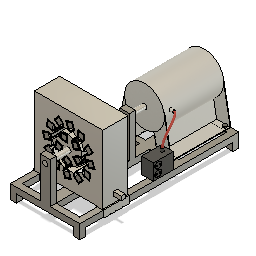
bannon_maher_magnetic_repulsion_motor_and_generator (Autodesk Fusion 360 design; units mm, degrees)
Autodesk Fusion 360 part; units mm, degrees
note: some values were not read from the file. Chosen so that the rebuilt part matches the saved one: which bodies a step acts on; which face or edge a step refers to. Set by a fixed rule: which sketch regions a step uses.
(part 1 of 2)
sketch "Sketch1" plane through (0, 0, 0) normal (0, 1, 0) x (1, 0, 0)
  line L0 (175, -400) -> (-175, -400)
  line L1 (-175, -400) -> (-175, 400)
  line L2 (-175, 400) -> (175, 400)
  line L3 (175, 400) -> (175, -400)
  line L4 (175, -400) -> (-175, 400) construction
  line L5 (-175, -400) -> (175, 400) construction
  line L6 (-145, -370) -> (-145, 370)
  line L7 (-145, 370) -> (145, 370)
  line L8 (145, 370) -> (145, -370)
  line L9 (145, -370) -> (-145, -370)
  dimension "d1" = 350
  dimension "d2" = 800
  dimension "d3" = 30
  measures "d1" distance of L1.end L2.end
  measures "d2" distance of L0.start L2.end
extrude "Extrude1" add sketch "Sketch1" along normal blind 30 makes body 1
sketch "Sketch2" plane through (0, 0, 0) normal (0, 1, 0) x (1, 0, 0)
  line L0 (-25, 370) -> (25, 370)
  line L1 (25, 370) -> (25, -370)
  line L2 (25, -370) -> (-25, -370)
  line L3 (-25, -370) -> (-25, 370)
  line L4 (-145, 370) -> (145, 370)
  line L5 (145, -370) -> (-145, -370)
  line L6 (0, 0) -> (0, 92.5114)
  dimension "d6" = 50
  measures "d6" distance of L1 L3
extrude "Extrude2" add sketch "Sketch2" along normal up to surface (30 mm away) bodies 1
ref_plane "WorkPlane1" through (0, 15, 400) normal (0, 0, -1) x (-1, 0, 0)
sketch "Sketch16" plane through (0, 0, 0) normal (0, -1, 0) x (1, 0, 0)
  line L0 (-25, -370) -> (-145, -370)
  line L1 (-145, -370) -> (-145, 370)
  line L2 (-145, 370) -> (-25, 370)
  line L3 (-25, 370) -> (-25, -370)
  line L4 (25, -370) -> (25, 370)
  line L5 (25, 370) -> (145, 370)
  line L6 (145, 370) -> (145, -370)
  line L7 (145, -370) -> (25, -370)
  line L8 (-175, -400) -> (175, -400)
  line L9 (175, -400) -> (175, 400)
  line L10 (175, 400) -> (-175, 400)
  line L11 (-175, 400) -> (-175, -400)
  line L12 (-175, 400) -> (-145, 400)
  line L13 (-145, 400) -> (-145, 370)
  line L14 (-145, 370) -> (-175, 370)
  line L15 (-175, 370) -> (-175, 400)
  line L16 (145, 370) -> (175, 370)
  line L17 (175, 370) -> (175, 400)
  line L18 (175, 400) -> (145, 400)
  line L19 (145, 400) -> (145, 370)
  line L20 (-145, -370) -> (-175, -370)
  line L21 (-175, -370) -> (-175, -400)
  line L22 (-175, -400) -> (-145, -400)
  line L23 (-145, -400) -> (-145, -370)
  line L24 (145, -370) -> (175, -370)
  line L25 (175, -370) -> (175, -400)
  line L26 (175, -400) -> (145, -400)
  line L27 (145, -400) -> (145, -370)
extrude "Extrude24" add sketch "Sketch16" along normal blind 40 contours L8 L11 L20 L21 L22 L23 | L10 L11 L12 L13 L14 L15 | L8 L9 L24 L25 L26 L27 | L9 L10 L16 L17 L18 L19 bodies 1
sketch "Sketch3" plane through (-92.5, 15, 400) normal (0, 0, -1) x (1, 0, 0)
  line L0 (117.5, -15) -> (237.5, -15)
  line L1 (237.5, -15) -> (117.5, -15)
  line L2 (67.5, -15) -> (-52.5, -15)
  line L3 (-52.5, -15) -> (67.5, -15)
  line L4 (267.5, -15) -> (-82.5, -15)
  line L5 (-82.5, -15) -> (267.5, -15)
  line L6 (117.5, -15) -> (67.5, -15)
  line L7 (67.5, -15) -> (67.5, -220)
  line L8 (67.5, -220) -> (117.5, -220)
  line L9 (117.5, -220) -> (117.5, -15)
  circle A0 centre (92.5, -190) radius 12.5
  line L10 (92.5, -190) -> (92.5, -220)
  dimension "d11" = 25
  dimension "d12" = 30
  dimension "d24" = 175
  measures "d11" diameter of A0
  measures "d12" distance of A0.centre L10.end
  measures "d24" distance of L2.start A0.centre
extrude "Extrude3" add sketch "Sketch3" along normal blind 30 separate body makes body 2
pattern_linear "R-Pattern1" count 2 spacing 400 along (0, 0, -1) of bodies 2 makes body 3
sketch "Sketch4" plane through (0, 0, 400) normal (0, 0, 1) x (1, 0, 0)
  circle A0 centre (0, 205) radius 12.5
  line L0 (25, 30) -> (25, 235)
  line L1 (25, 235) -> (-25, 235)
  line L2 (-25, 235) -> (-25, 30)
  line L3 (-25, 30) -> (25, 30)
extrude "Extrude4" add sketch "Sketch4" along normal blind 0 and the other way blind 500 separate body contours A0 makes body 4
sketch "Sketch5" plane through (0, 0, -100) normal (0, 0, -1) x (-1, 0, 0)
  circle A0 centre (0, 205) radius 12.5
  circle A1 centre (0, 205) radius 100
  dimension "d23" = 200
  measures "d23" diameter of A1
extrude "Extrude5" add sketch "Sketch5" along normal up to surface (300 mm away) separate body contours A0 | A1 makes body 5
ref_plane "WorkPlane2" through (0, 132.5, 185) normal (0, 0, -1) x (1, 0, 0)
sketch "Sketch6" plane through (0, 120, 185) normal (0, 0, -1) x (1, 0, 0)
  line L0 (-175, 90) -> (175, 90)
  line L1 (175, 90) -> (175, -260)
  line L2 (175, -260) -> (-175, -260)
  line L3 (-175, -260) -> (-175, 90)
  point P0 (-175, 90)
  point P1 (175, 90)
  dimension "d27" = 350
  measures "d27" distance of P1 L1.end
extrude "Extrude6" add sketch "Sketch6" along normal mid plane 200 separate body makes body 6
shell "Shell1" thickness 3 removed faces 0 bodies 6
split "Split1" by plane through (0, 132.5, 185) normal (0, 0, -1) bodies 6 makes body 7 at (58.3333, 263.3333, 85)
sketch "Sketch7" plane through (0, 30, 0) normal (0, 1, 0) x (-1, 0, 0)
  line L0 (-25, -370) -> (-145, -370)
  line L1 (-145, -370) -> (-145, 370)
  line L2 (-145, 370) -> (-25, 370)
  line L3 (-25, 370) -> (-25, -370)
  line L4 (25, -370) -> (25, 370)
  line L5 (25, 370) -> (145, 370)
  line L6 (145, 370) -> (145, -370)
  line L7 (145, -370) -> (25, -370)
  line L8 (-175, -400) -> (175, -400)
  line L9 (175, -400) -> (175, 400)
  line L10 (175, 400) -> (-175, 400)
  line L11 (-175, 400) -> (-175, -400)
  line L12 (-175, -70) -> (-115, -70)
  line L13 (-115, -70) -> (-115, 30)
  line L14 (-115, 30) -> (-175, 30)
  line L15 (-175, 30) -> (-175, -70)
  point P0 (-100, -100)
  dimension "d31" = 60
  dimension "d32" = 100
  dimension "d175" = 30
  measures "d31" distance of L13.end L14.end
  measures "d32" distance of L12.end L13.end
  measures "d175" distance of L12 P0
extrude "Extrude7" add sketch "Sketch7" along normal blind 80 separate body contours L1 L11 L12 L14 L15 | L1 L12 L13 L14 makes body 8
sketch "Sketch8" plane through (0, 0, 282) normal (0, 0, -1) x (-1, 0, 0)
  line L0 (172, 377) -> (-172, 377)
  line L1 (-172, 377) -> (-172, 33)
  line L2 (-172, 33) -> (172, 33)
  line L3 (172, 33) -> (172, 377)
  circle A0 centre (0, 205) radius 12.5
  line L4 (-15.4979, 331.8655) -> (-24.1853, 307.9973)
  line L5 (-24.1853, 307.9973) -> (-0.3171, 299.31)
  line L6 (-0.3171, 299.31) -> (8.3702, 323.1782)
  line L7 (8.3702, 323.1782) -> (-15.4979, 331.8655)
  line L8 (0, 205) -> (0, 253.0629)
  line L9 (-24.1853, 307.9973) -> (-19.6858, 297.8462)
  line L10 (-19.6858, 297.8462) -> (-10.2889, 294.426)
  line L11 (-10.2889, 294.426) -> (-0.3171, 299.31)
  line L12 (-29.573, 307.8136) -> (-23.3949, 293.8753)
  line L13 (-23.3949, 293.8753) -> (-10, 289)
  line L14 (-10, 289) -> (3.6921, 295.7061)
  line L15 (3.6921, 295.7061) -> (14.7788, 326.1666)
  line L16 (14.7788, 326.1666) -> (-18.4863, 338.2741)
  line L17 (-18.4863, 338.2741) -> (-29.573, 307.8136)
  line L18 (-35.2399, 283.2881) -> (0.5993, 270.2437)
  line L19 (-32.9714, 267.5639) -> (-19.5766, 262.6886)
  line L20 (-19.5766, 262.6886) -> (-13.3984, 248.7503)
  line L21 (-13.3984, 248.7503) -> (-24.4851, 218.2899)
  line L22 (-18.7862, 248.5666) -> (-27.4735, 224.6984)
  line L23 (-24.4851, 218.2899) -> (-57.7502, 230.3974)
  line L24 (-57.7502, 230.3974) -> (-46.6635, 260.8578)
  line L25 (-51.3417, 233.3857) -> (-42.6543, 257.2539)
  line L26 (-27.4735, 224.6984) -> (-51.3417, 233.3857)
  line L27 (-42.6543, 257.2539) -> (-32.6826, 262.1379)
  line L28 (-32.6826, 262.1379) -> (-23.2856, 258.7177)
  line L29 (-23.2856, 258.7177) -> (-18.7862, 248.5666)
  line L30 (-46.6635, 260.8578) -> (-32.9714, 267.5639)
  line L31 (-10.2889, 294.426) -> (-10, 289)
  line L32 (-19.6858, 297.8462) -> (-23.3949, 293.8753)
  line L33 (-23.2856, 258.7177) -> (-19.5766, 262.6886)
  line L34 (-32.6826, 262.1379) -> (-32.9714, 267.5639)
  line L35 (-64.6982, 270.2709) -> (-50.6603, 272.7461)
  line L36 (-50.6603, 272.7461) -> (-42.1556, 285.3999)
  line L37 (-53.6234, 277.3008) -> (-47.4296, 286.5163)
  line L38 (-63.4715, 275.5643) -> (-53.6234, 277.3008)
  line L39 (-53.6234, 277.3008) -> (-50.6603, 272.7461)
  line L40 (-63.4715, 275.5643) -> (-64.6982, 270.2709)
  line L41 (-77.0178, 279.2527) -> (-64.6982, 270.2709)
  line L42 (-72.4437, 282.1057) -> (-63.4715, 275.5643)
  line L43 (-76.8544, 307.1198) -> (-72.4437, 282.1057)
  line L44 (-82.6467, 311.1756) -> (-77.0178, 279.2527)
  line L45 (-47.4296, 286.5163) -> (-51.8403, 311.5304)
  line L46 (-42.1556, 285.3999) -> (-47.7845, 317.3227)
  line L47 (-47.7845, 317.3227) -> (-82.6467, 311.1756)
  line L48 (-51.8403, 311.5304) -> (-76.8544, 307.1198)
  line L49 (-88.6657, 229.1771) -> (-77.7461, 238.3397)
  line L50 (-77.7461, 238.3397) -> (-76.7078, 253.5505)
  line L51 (-82.5896, 240.8026) -> (-81.8334, 251.8804)
  line L52 (-90.2501, 234.3747) -> (-82.5896, 240.8026)
  line L53 (-82.5896, 240.8026) -> (-77.7461, 238.3397)
  line L54 (-90.2501, 234.3747) -> (-88.6657, 229.1771)
  line L55 (-103.8257, 230.7958) -> (-88.6657, 229.1771)
  line L56 (-101.2909, 235.5536) -> (-90.2501, 234.3747)
  line L57 (-117.6177, 255.0111) -> (-101.2909, 235.5536)
  line L58 (-124.6619, 255.6274) -> (-103.8257, 230.7958)
  line L59 (-81.8334, 251.8804) -> (-98.1602, 271.3379)
  line L60 (-76.7078, 253.5505) -> (-97.5439, 278.3821)
  line L61 (-97.5439, 278.3821) -> (-124.6619, 255.6274)
  line L62 (-98.1602, 271.3379) -> (-117.6177, 255.0111)
  line L63 (-88.8753, 181.6051) -> (-84, 195)
  line L64 (-84, 195) -> (-90.7061, 208.6921)
  line L65 (-89.426, 194.7111) -> (-94.31, 204.6829)
  line L66 (-92.8462, 185.3142) -> (-89.426, 194.7111)
  line L67 (-89.426, 194.7111) -> (-84, 195)
  line L68 (-92.8462, 185.3142) -> (-88.8753, 181.6051)
  line L69 (-102.8136, 175.427) -> (-88.8753, 181.6051)
  line L70 (-102.9973, 180.8147) -> (-92.8462, 185.3142)
  line L71 (-126.8655, 189.5021) -> (-102.9973, 180.8147)
  line L72 (-133.2741, 186.5137) -> (-102.8136, 175.427)
  line L73 (-94.31, 204.6829) -> (-118.1782, 213.3702)
  line L74 (-90.7061, 208.6921) -> (-121.1666, 219.7788)
  line L75 (-121.1666, 219.7788) -> (-133.2741, 186.5137)
  line L76 (-118.1782, 213.3702) -> (-126.8655, 189.5021)
  line L77 (-65.2709, 140.3018) -> (-67.7461, 154.3397)
  line L78 (-67.7461, 154.3397) -> (-80.3999, 162.8444)
  line L79 (-72.3008, 151.3766) -> (-81.5163, 157.5704)
  line L80 (-70.5643, 141.5285) -> (-72.3008, 151.3766)
  line L81 (-72.3008, 151.3766) -> (-67.7461, 154.3397)
  line L82 (-70.5643, 141.5285) -> (-65.2709, 140.3018)
  line L83 (-74.2527, 127.9822) -> (-65.2709, 140.3018)
  line L84 (-77.1057, 132.5563) -> (-70.5643, 141.5285)
  line L85 (-102.1198, 128.1456) -> (-77.1057, 132.5563)
  line L86 (-106.1756, 122.3533) -> (-74.2527, 127.9822)
  line L87 (-81.5163, 157.5704) -> (-106.5304, 153.1597)
  line L88 (-80.3999, 162.8444) -> (-112.3227, 157.2155)
  line L89 (-112.3227, 157.2155) -> (-106.1756, 122.3533)
  line L90 (-106.5304, 153.1597) -> (-102.1198, 128.1456)
  line L91 (-24.1771, 116.3343) -> (-33.3397, 127.2539)
  line L92 (-33.3397, 127.2539) -> (-48.5505, 128.2922)
  line L93 (-35.8026, 122.4104) -> (-46.8804, 123.1666)
  line L94 (-29.3747, 114.7499) -> (-35.8026, 122.4104)
  line L95 (-35.8026, 122.4104) -> (-33.3397, 127.2539)
  line L96 (-29.3747, 114.7499) -> (-24.1771, 116.3343)
  line L97 (-25.7958, 101.1743) -> (-24.1771, 116.3343)
  line L98 (-30.5536, 103.7091) -> (-29.3747, 114.7499)
  line L99 (-50.0111, 87.3823) -> (-30.5536, 103.7091)
  line L100 (-50.6274, 80.3381) -> (-25.7958, 101.1743)
  line L101 (-46.8804, 123.1666) -> (-66.3379, 106.8398)
  line L102 (-48.5505, 128.2922) -> (-73.3821, 107.4561)
  line L103 (-73.3821, 107.4561) -> (-50.6274, 80.3381)
  line L104 (-66.3379, 106.8398) -> (-50.0111, 87.3823)
  line L105 (23.3949, 116.1247) -> (10, 121)
  line L106 (10, 121) -> (-3.6921, 114.2939)
  line L107 (10.2889, 115.574) -> (0.3171, 110.69)
  line L108 (19.6858, 112.1538) -> (10.2889, 115.574)
  line L109 (10.2889, 115.574) -> (10, 121)
  line L110 (19.6858, 112.1538) -> (23.3949, 116.1247)
  line L111 (29.573, 102.1864) -> (23.3949, 116.1247)
  line L112 (24.1853, 102.0027) -> (19.6858, 112.1538)
  line L113 (15.4979, 78.1345) -> (24.1853, 102.0027)
  line L114 (18.4863, 71.7259) -> (29.573, 102.1864)
  line L115 (0.3171, 110.69) -> (-8.3702, 86.8218)
  line L116 (-3.6921, 114.2939) -> (-14.7788, 83.8334)
  line L117 (-14.7788, 83.8334) -> (18.4863, 71.7259)
  line L118 (-8.3702, 86.8218) -> (15.4979, 78.1345)
  line L119 (64.6982, 139.7291) -> (50.6603, 137.2539)
  line L120 (50.6603, 137.2539) -> (42.1556, 124.6001)
  line L121 (53.6234, 132.6992) -> (47.4296, 123.4837)
  line L122 (63.4715, 134.4357) -> (53.6234, 132.6992)
  line L123 (53.6234, 132.6992) -> (50.6603, 137.2539)
  line L124 (63.4715, 134.4357) -> (64.6982, 139.7291)
  line L125 (77.0178, 130.7473) -> (64.6982, 139.7291)
  line L126 (72.4437, 127.8943) -> (63.4715, 134.4357)
  line L127 (76.8544, 102.8802) -> (72.4437, 127.8943)
  line L128 (82.6467, 98.8244) -> (77.0178, 130.7473)
  line L129 (47.4296, 123.4837) -> (51.8403, 98.4696)
  line L130 (42.1556, 124.6001) -> (47.7845, 92.6773)
  line L131 (47.7845, 92.6773) -> (82.6467, 98.8244)
  line L132 (51.8403, 98.4696) -> (76.8544, 102.8802)
  line L133 (88.6657, 180.8229) -> (77.7461, 171.6603)
  line L134 (77.7461, 171.6603) -> (76.7078, 156.4495)
  line L135 (82.5896, 169.1974) -> (81.8334, 158.1196)
  line L136 (90.2501, 175.6253) -> (82.5896, 169.1974)
  line L137 (82.5896, 169.1974) -> (77.7461, 171.6603)
  line L138 (90.2501, 175.6253) -> (88.6657, 180.8229)
  line L139 (103.8257, 179.2042) -> (88.6657, 180.8229)
  line L140 (101.2909, 174.4464) -> (90.2501, 175.6253)
  line L141 (117.6177, 154.9889) -> (101.2909, 174.4464)
  line L142 (124.6619, 154.3726) -> (103.8257, 179.2042)
  line L143 (81.8334, 158.1196) -> (98.1602, 138.6621)
  line L144 (76.7078, 156.4495) -> (97.5439, 131.6179)
  line L145 (97.5439, 131.6179) -> (124.6619, 154.3726)
  line L146 (98.1602, 138.6621) -> (117.6177, 154.9889)
  line L147 (88.8753, 228.3949) -> (84, 215)
  line L148 (84, 215) -> (90.7061, 201.3079)
  line L149 (89.426, 215.2889) -> (94.31, 205.3171)
  line L150 (92.8462, 224.6858) -> (89.426, 215.2889)
  line L151 (89.426, 215.2889) -> (84, 215)
  line L152 (92.8462, 224.6858) -> (88.8753, 228.3949)
  line L153 (102.8136, 234.573) -> (88.8753, 228.3949)
  line L154 (102.9973, 229.1853) -> (92.8462, 224.6858)
  line L155 (126.8655, 220.4979) -> (102.9973, 229.1853)
  line L156 (133.2741, 223.4863) -> (102.8136, 234.573)
  line L157 (94.31, 205.3171) -> (118.1782, 196.6298)
  line L158 (90.7061, 201.3079) -> (121.1666, 190.2212)
  line L159 (121.1666, 190.2212) -> (133.2741, 223.4863)
  line L160 (118.1782, 196.6298) -> (126.8655, 220.4979)
  line L161 (65.2709, 269.6982) -> (67.7461, 255.6603)
  line L162 (67.7461, 255.6603) -> (80.3999, 247.1556)
  line L163 (72.3008, 258.6234) -> (81.5163, 252.4296)
  line L164 (70.5643, 268.4715) -> (72.3008, 258.6234)
  line L165 (72.3008, 258.6234) -> (67.7461, 255.6603)
  line L166 (70.5643, 268.4715) -> (65.2709, 269.6982)
  line L167 (74.2527, 282.0178) -> (65.2709, 269.6982)
  line L168 (77.1057, 277.4437) -> (70.5643, 268.4715)
  line L169 (102.1198, 281.8544) -> (77.1057, 277.4437)
  line L170 (106.1756, 287.6467) -> (74.2527, 282.0178)
  line L171 (81.5163, 252.4296) -> (106.5304, 256.8403)
  line L172 (80.3999, 247.1556) -> (112.3227, 252.7845)
  line L173 (112.3227, 252.7845) -> (106.1756, 287.6467)
  line L174 (106.5304, 256.8403) -> (102.1198, 281.8544)
  line L175 (24.1771, 293.6657) -> (33.3397, 282.7461)
  line L176 (33.3397, 282.7461) -> (48.5505, 281.7078)
  line L177 (35.8026, 287.5896) -> (46.8804, 286.8334)
  line L178 (29.3747, 295.2501) -> (35.8026, 287.5896)
  line L179 (35.8026, 287.5896) -> (33.3397, 282.7461)
  line L180 (29.3747, 295.2501) -> (24.1771, 293.6657)
  line L181 (25.7958, 308.8257) -> (24.1771, 293.6657)
  line L182 (30.5536, 306.2909) -> (29.3747, 295.2501)
  line L183 (50.0111, 322.6177) -> (30.5536, 306.2909)
  line L184 (50.6274, 329.6619) -> (25.7958, 308.8257)
  line L185 (46.8804, 286.8334) -> (66.3379, 303.1602)
  line L186 (48.5505, 281.7078) -> (73.3821, 302.5439)
  line L187 (73.3821, 302.5439) -> (50.6274, 329.6619)
  line L188 (66.3379, 303.1602) -> (50.0111, 322.6177)
  line L189 (-20.2057, 185.8201) -> (-42.0001, 157.9245)
  line L190 (-45.7493, 205.7769) -> (-20.2057, 185.8201)
  line L191 (-60.9146, 204.2083) -> (-45.7493, 205.7769)
  line L192 (-69.6906, 192.9756) -> (-60.9146, 204.2083)
  line L193 (-67.5438, 177.8814) -> (-69.6906, 192.9756)
  line L194 (-42.0001, 157.9245) -> (-67.5438, 177.8814)
  line L195 (-42.8619, 164.9429) -> (-62.8774, 180.5807)
  line L196 (-27.2241, 184.9583) -> (-42.8619, 164.9429)
  line L197 (-47.2396, 200.5961) -> (-27.2241, 184.9583)
  line L198 (-58.2842, 199.4537) -> (-47.2396, 200.5961)
  line L199 (-64.4408, 191.5736) -> (-58.2842, 199.4537)
  line L200 (-62.8774, 180.5807) -> (-64.4408, 191.5736)
  line L201 (-64.4408, 191.5736) -> (-69.6906, 192.9756)
  line L202 (-58.2842, 199.4537) -> (-60.9146, 204.2083)
  line L203 (11.9973, 179.8563) -> (31.7927, 150.5084)
  line L204 (-14.8762, 161.7299) -> (11.9973, 179.8563)
  line L205 (-18.0707, 146.8221) -> (-14.8762, 161.7299)
  line L206 (-10.0997, 135.0046) -> (-18.0707, 146.8221)
  line L207 (4.9192, 132.3819) -> (-10.0997, 135.0046)
  line L208 (31.7927, 150.5084) -> (4.9192, 132.3819)
  line L209 (24.8516, 151.8576) -> (3.794, 137.6541)
  line L210 (10.6481, 172.9151) -> (24.8516, 151.8576)
  line L211 (-10.4095, 158.7116) -> (10.6481, 172.9151)
  line L212 (-12.736, 147.8545) -> (-10.4095, 158.7116)
  line L213 (-7.1441, 139.5641) -> (-12.736, 147.8545)
  line L214 (3.794, 137.6541) -> (-7.1441, 139.5641)
  line L215 (-7.1441, 139.5641) -> (-10.0997, 135.0046)
  line L216 (-12.736, 147.8545) -> (-18.0707, 146.8221)
  line L217 (27.6204, 208.6403) -> (61.6491, 218.3978)
  line L218 (36.5553, 177.4807) -> (27.6204, 208.6403)
  line L219 (49.7463, 169.8358) -> (36.5553, 177.4807)
  line L220 (63.4486, 173.7648) -> (49.7463, 169.8358)
  line L221 (70.584, 187.2382) -> (63.4486, 173.7648)
  line L222 (61.6491, 218.3978) -> (70.584, 187.2382)
  line L223 (58.221, 212.2133) -> (65.2222, 187.7973)
  line L224 (33.8049, 205.2121) -> (58.221, 212.2133)
  line L225 (40.8061, 180.7961) -> (33.8049, 205.2121)
  line L226 (50.4129, 175.2284) -> (40.8061, 180.7961)
  line L227 (60.0256, 177.9848) -> (50.4129, 175.2284)
  line L228 (65.2222, 187.7973) -> (60.0256, 177.9848)
  line L229 (60.0256, 177.9848) -> (63.4486, 173.7648)
  line L230 (50.4129, 175.2284) -> (49.7463, 169.8358)
  line L231 (5.0731, 232.3935) -> (6.3085, 267.7719)
  line L232 (37.4687, 231.2622) -> (5.0731, 232.3935)
  line L233 (48.8156, 241.4452) -> (37.4687, 231.2622)
  line L234 (49.3131, 255.691) -> (48.8156, 241.4452)
  line L235 (38.7041, 266.6407) -> (49.3131, 255.691)
  line L236 (6.3085, 267.7719) -> (38.7041, 266.6407)
  line L237 (11.131, 262.6005) -> (36.5155, 261.714)
  line L238 (10.2445, 237.216) -> (11.131, 262.6005)
  line L239 (35.6291, 236.3295) -> (10.2445, 237.216)
  line L240 (43.8929, 243.7456) -> (35.6291, 236.3295)
  line L241 (44.2419, 253.7395) -> (43.8929, 243.7456)
  line L242 (36.5155, 261.714) -> (44.2419, 253.7395)
  line L243 (44.2419, 253.7395) -> (49.3131, 255.691)
  line L244 (43.8929, 243.7456) -> (48.8156, 241.4452)
  line L245 (-46.6635, 260.8578) -> (-69.5531, 249.6469)
  line L246 (-69.5531, 249.6469) -> (-60.9146, 204.2083)
  line L247 (-23.3949, 293.8753) -> (-50.6603, 272.7461)
  line L248 (-64.6982, 270.2709) -> (-77.7461, 238.3397)
  line L249 (-88.6657, 229.1771) -> (-84, 195)
  line L250 (-88.8753, 181.6051) -> (-67.7461, 154.3397)
  line L251 (-65.2709, 140.3018) -> (-33.3397, 127.2539)
  line L252 (-24.1771, 116.3343) -> (10, 121)
  line L253 (23.3949, 116.1247) -> (50.6603, 137.2539)
  line L254 (64.6982, 139.7291) -> (77.7461, 171.6603)
  line L255 (88.6657, 180.8229) -> (84, 215)
  line L256 (88.8753, 228.3949) -> (67.7461, 255.6603)
  line L257 (65.2709, 269.6982) -> (33.3397, 282.7461)
  line L258 (24.1771, 293.6657) -> (-10, 289)
  line L259 (-67.5438, 177.8814) -> (-63.9549, 152.6477)
  line L260 (-63.9549, 152.6477) -> (-18.0707, 146.8221)
  line L261 (4.9192, 132.3819) -> (30.0268, 127.9976)
  line L262 (30.0268, 127.9976) -> (49.7463, 169.8358)
  line L263 (70.584, 187.2382) -> (82.5125, 209.7622)
  line L264 (82.5125, 209.7622) -> (48.8156, 241.4452)
  line L265 (38.7041, 266.6407) -> (20.9687, 284.9456)
  line L266 (20.9687, 284.9456) -> (-19.5766, 262.6886)
  circle A1 centre (0, 205) radius 12.5
  line L267 (32.6835, 272.8546) -> (0.9606, 273.9624)
  line L268 (-57.7502, 230.3974) -> (-46.6635, 260.8578)
  line L269 (-42.0001, 157.9245) -> (-67.5438, 177.8814)
  line L270 (31.7927, 150.5084) -> (4.9192, 132.3819)
  line L271 (61.6491, 218.3978) -> (70.584, 187.2382)
  line L272 (-54.4338, 257.0521) -> (-65.2902, 227.2242)
  line L273 (-66.3255, 169.3154) -> (-41.3122, 149.7729)
  line L274 (13.4424, 130.8936) -> (39.7579, 148.6436)
  line L275 (74.6333, 194.8843) -> (65.884, 225.3969)
  dimension "d35" = 20
  dimension "d36" = 5
  dimension "d37" = 25.4
  dimension "d38" = 25.4
  dimension "d39" = 10
  dimension "d40" = 8
  dimension "d41" = 84
  dimension "d42" = 10
  dimension "d43" = 14
  dimension "d45" = 360
  dimension "d47" = 360
  dimension "d48" = 8
  dimension "d50" = 360
  dimension "d52" = 360
  dimension "d123" = 6
  dimension "d125" = 360
  dimension "d127" = 360
  measures "d35" angle of L6 L8
  measures "d37" distance of L4.start L6.end
  measures "d38" distance of L5.end L6.end
  measures "d39" distance of L9.end L10.end
  measures "d40" distance of L5 L10
  measures "d41" distance of A0.centre L13.end
  measures "d42" distance of L8 L13.end
  measures "d43" distance of L13 L18
  measures "d48" distance of L23.end L246
  measures "d123" distance of L236 L267
extrude "Extrude8" add sketch "Sketch8" along normal blind 127 separate body contours L0 L1 L2 L3 makes body 9
extrude "Extrude9" add sketch "Sketch8" along normal blind 127 separate body contours L4 L6 L7 L9 L11 L12 L14 L15 L16 L17 L31 L32 | L36 L37 L39 L40 L41 L42 L43 L44 L45 L46 L47 L48 | L176 L177 L179 L180 L181 L182 L183 L184 L185 L186 L187 L188 | L50 L51 L53 L54 L55 L56 L57 L58 L59 L60 L61 L62 | L162 L163 L165 L166 L167 L168 L169 L170 L171 L172 L173 L174 | L64 L65 L67 L68 L69 L70 L71 L72 L73 L74 L75 L76 | L148 L149 L151 L152 L153 L154 L155 L156 L157 L158 L159 L160 | L78 L79 L81 L82 L83 L84 L85 L86 L87 L88 L89 L90 | L134 L135 L137 L138 L139 L140 L141 L142 L143 L144 L145 L146 | L92 L93 L95 L96 L97 L98 L99 L100 L101 L102 L103 L104 | L120 L121 L123 L124 L125 L126 L127 L128 L129 L130 L131 L132 | L106 L107 L109 L110 L111 L112 L113 L114 L115 L116 L117 L118 | L20 L21 L22 L23 L24 L25 L26 L27 L29 L30 L33 L34 L268 | L189 L190 L191 L193 L194 L195 L196 L197 L198 L200 L201 L202 L269 | L231 L232 L233 L235 L236 L237 L238 L239 L240 L242 L243 L244 | L203 L204 L205 L207 L208 L209 L210 L211 L212 L214 L215 L216 L270 | L217 L218 L219 L221 L222 L223 L224 L225 L226 L228 L229 L230 L271 makes body 10 at (-125.2024, 201.3096, 239.6667) makes body 11 at (65.7972, 98.4168, 239.6667) makes body 12 at (59.4052, 315.2737, 239.6667) makes body 13 at (106.5832, 270.7972, 239.6667) makes body 14 at (3.6904, 79.7976, 239.6667) makes body 15 at (-110.2737, 264.4052, 239.6667) makes body 16 at (-106.5832, 139.2028, 239.6667) makes body 17 at (110.2737, 145.5948, 239.6667) makes body 18 at (-3.6904, 330.2024, 239.6667) makes body 19 at (125.2024, 208.6904, 239.6667) makes body 20 at (-59.4052, 94.7263, 239.6667) makes body 21 at (-65.7972, 311.5832, 239.6667) makes body 22 at (27.4705, 176.5215, 239.6667) makes body 23 at (35.5735, 222.3257, 239.6667) makes body 24 at (-18.5958, 170.0737, 239.6667) makes body 25 at (-5.4849, 244.1863, 239.6667) makes body 26 at (-38.9633, 211.8928, 239.6667)
extrude "Extrude10" add sketch "Sketch8" along normal blind 127 separate body contours L4 L5 L6 L7 | L5 L9 L10 L11 | L37 L38 L42 L43 L45 L48 | L177 L178 L182 L183 L185 L188 | L51 L52 L56 L57 L59 L62 | L163 L164 L168 L169 L171 L174 | L65 L66 L70 L71 L73 L76 | L149 L150 L154 L155 L157 L160 | L79 L80 L84 L85 L87 L90 | L135 L136 L140 L141 L143 L146 | L93 L94 L98 L99 L101 L104 | L121 L122 L126 L127 L129 L132 | L107 L108 L112 L113 L115 L118 | L22 L25 L26 L27 L28 L29 | L195 L196 L197 L198 L199 L200 | L237 L238 L239 L240 L241 L242 | L209 L210 L211 L212 L213 L214 | L223 L224 L225 L226 L227 L228 makes body 27 at (-121.074, 204.5858, 197.3333) makes body 28 at (0.4142, 83.926, 197.3333) makes body 29 at (60.1783, 310.0602, 197.3333) makes body 30 at (32.4367, 178.2865, 239.6667) makes body 31 at (-15.3826, 165.896, 197.3333) makes body 32 at (-0.4142, 326.074, 197.3333) makes body 33 at (60.8957, 100.354, 197.3333) makes body 34 at (-104.646, 144.1043, 239.6667) makes body 35 at (-105.0602, 265.1783, 239.6667) makes body 36 at (105.0602, 144.8217, 197.3333) makes body 37 at (104.646, 265.8957, 239.6667) makes body 38 at (35.4295, 227.5942, 197.3333) makes body 39 at (-41.9436, 207.5459, 239.6667) makes body 40 at (-10.54, 245.6775, 197.3333) makes body 41 at (121.074, 205.4142, 197.3333) makes body 42 at (-60.1783, 99.9398, 239.6667) makes body 43 at (-60.8957, 309.646, 239.6667)
sketch "Sketch13" plane through (0, 0, 282) normal (0, 0, 1) x (1, 0, 0)
  line L0 (-24.1771, 293.6657) -> (10, 289)
  line L1 (10, 289) -> (-3.6921, 295.7061)
  line L2 (-3.6921, 295.7061) -> (-14.7788, 326.1666)
  line L3 (-14.7788, 326.1666) -> (18.4863, 338.2741)
  line L4 (18.4863, 338.2741) -> (29.573, 307.8136)
  line L5 (29.573, 307.8136) -> (23.3949, 293.8753)
  line L6 (23.3949, 293.8753) -> (50.6603, 272.7461)
  line L7 (50.6603, 272.7461) -> (42.1556, 285.3999)
  line L8 (42.1556, 285.3999) -> (47.7845, 317.3227)
  line L9 (47.7845, 317.3227) -> (82.6467, 311.1756)
  line L10 (82.6467, 311.1756) -> (77.0178, 279.2527)
  line L11 (77.0178, 279.2527) -> (64.6982, 270.2709)
  line L12 (64.6982, 270.2709) -> (77.7461, 238.3397)
  line L13 (77.7461, 238.3397) -> (76.7078, 253.5505)
  line L14 (76.7078, 253.5505) -> (97.5439, 278.3821)
  line L15 (97.5439, 278.3821) -> (124.6619, 255.6274)
  line L16 (124.6619, 255.6274) -> (103.8257, 230.7958)
  line L17 (103.8257, 230.7958) -> (88.6657, 229.1771)
  line L18 (88.6657, 229.1771) -> (84, 195)
  line L19 (84, 195) -> (90.7061, 208.6921)
  line L20 (90.7061, 208.6921) -> (121.1666, 219.7788)
  line L21 (121.1666, 219.7788) -> (133.2741, 186.5137)
  line L22 (133.2741, 186.5137) -> (102.8136, 175.427)
  line L23 (102.8136, 175.427) -> (88.8753, 181.6051)
  line L24 (88.8753, 181.6051) -> (67.7461, 154.3397)
  line L25 (67.7461, 154.3397) -> (80.3999, 162.8444)
  line L26 (80.3999, 162.8444) -> (112.3227, 157.2155)
  line L27 (112.3227, 157.2155) -> (106.1756, 122.3533)
  line L28 (106.1756, 122.3533) -> (74.2527, 127.9822)
  line L29 (74.2527, 127.9822) -> (65.2709, 140.3018)
  line L30 (65.2709, 140.3018) -> (33.3397, 127.2539)
  line L31 (33.3397, 127.2539) -> (48.5505, 128.2922)
  line L32 (48.5505, 128.2922) -> (73.3821, 107.4561)
  line L33 (73.3821, 107.4561) -> (50.6274, 80.3381)
  line L34 (50.6274, 80.3381) -> (25.7958, 101.1743)
  line L35 (25.7958, 101.1743) -> (24.1771, 116.3343)
  line L36 (24.1771, 116.3343) -> (-10, 121)
  line L37 (-10, 121) -> (3.6921, 114.2939)
  line L38 (3.6921, 114.2939) -> (14.7788, 83.8334)
  line L39 (14.7788, 83.8334) -> (-18.4863, 71.7259)
  line L40 (-18.4863, 71.7259) -> (-29.573, 102.1864)
  line L41 (-29.573, 102.1864) -> (-23.3949, 116.1247)
  line L42 (-23.3949, 116.1247) -> (-50.6603, 137.2539)
  line L43 (-50.6603, 137.2539) -> (-42.1556, 124.6001)
  line L44 (-42.1556, 124.6001) -> (-47.7845, 92.6773)
  line L45 (-47.7845, 92.6773) -> (-82.6467, 98.8244)
  line L46 (-82.6467, 98.8244) -> (-77.0178, 130.7473)
  line L47 (-77.0178, 130.7473) -> (-64.6982, 139.7291)
  line L48 (-64.6982, 139.7291) -> (-77.7461, 171.6603)
  line L49 (-77.7461, 171.6603) -> (-76.7078, 156.4495)
  line L50 (-76.7078, 156.4495) -> (-97.5439, 131.6179)
  line L51 (-97.5439, 131.6179) -> (-124.6619, 154.3726)
  line L52 (-124.6619, 154.3726) -> (-103.8257, 179.2042)
  line L53 (-103.8257, 179.2042) -> (-88.6657, 180.8229)
  line L54 (-88.6657, 180.8229) -> (-84, 215)
  line L55 (-84, 215) -> (-90.7061, 201.3079)
  line L56 (-90.7061, 201.3079) -> (-121.1666, 190.2212)
  line L57 (-121.1666, 190.2212) -> (-133.2741, 223.4863)
  line L58 (-133.2741, 223.4863) -> (-102.8136, 234.573)
  line L59 (-102.8136, 234.573) -> (-88.8753, 228.3949)
  line L60 (-88.8753, 228.3949) -> (-67.7461, 255.6603)
  line L61 (-67.7461, 255.6603) -> (-80.3999, 247.1556)
  line L62 (-80.3999, 247.1556) -> (-112.3227, 252.7845)
  line L63 (-112.3227, 252.7845) -> (-106.1756, 287.6467)
  line L64 (-106.1756, 287.6467) -> (-74.2527, 282.0178)
  line L65 (-74.2527, 282.0178) -> (-65.2709, 269.6982)
  line L66 (-65.2709, 269.6982) -> (-33.3397, 282.7461)
  line L67 (-33.3397, 282.7461) -> (-48.5505, 281.7078)
  line L68 (-48.5505, 281.7078) -> (-73.3821, 302.5439)
  line L69 (-73.3821, 302.5439) -> (-50.6274, 329.6619)
  line L70 (-50.6274, 329.6619) -> (-25.7958, 308.8257)
  line L71 (-25.7958, 308.8257) -> (-24.1771, 293.6657)
  line L72 (-172, 377) -> (-172, 33)
  line L73 (-172, 33) -> (172, 33)
  line L74 (172, 33) -> (172, 377)
  line L75 (172, 377) -> (-172, 377)
  line L76 (0.3171, 299.31) -> (10.2889, 294.426)
  line L77 (10.2889, 294.426) -> (19.6858, 297.8462)
  line L78 (19.6858, 297.8462) -> (24.1853, 307.9973)
  line L79 (24.1853, 307.9973) -> (15.4979, 331.8655)
  line L80 (15.4979, 331.8655) -> (-8.3702, 323.1782)
  line L81 (-8.3702, 323.1782) -> (0.3171, 299.31)
  line L82 (0.3171, 299.31) -> (24.1853, 307.9973)
  line L83 (32.6826, 262.1379) -> (23.2856, 258.7177)
  line L84 (23.2856, 258.7177) -> (18.7862, 248.5666)
  line L85 (18.7862, 248.5666) -> (27.4735, 224.6984)
  line L86 (27.4735, 224.6984) -> (51.3417, 233.3857)
  line L87 (51.3417, 233.3857) -> (42.6543, 257.2539)
  line L88 (42.6543, 257.2539) -> (32.6826, 262.1379)
  line L89 (18.7862, 248.5666) -> (42.6543, 257.2539)
  circle A0 centre (0, 205) radius 12.5
  line L90 (-35.8026, 287.5896) -> (-29.3747, 295.2501)
  line L91 (-29.3747, 295.2501) -> (-30.5536, 306.2909)
  line L92 (-46.8804, 286.8334) -> (-30.5536, 306.2909)
  line L93 (-46.8804, 286.8334) -> (-35.8026, 287.5896)
  line L94 (-72.3008, 258.6234) -> (-70.5643, 268.4715)
  line L95 (-70.5643, 268.4715) -> (-77.1057, 277.4437)
  line L96 (-81.5163, 252.4296) -> (-77.1057, 277.4437)
  line L97 (-81.5163, 252.4296) -> (-72.3008, 258.6234)
  line L98 (-89.426, 215.2889) -> (-92.8462, 224.6858)
  line L99 (-92.8462, 224.6858) -> (-102.9973, 229.1853)
  line L100 (-94.31, 205.3171) -> (-102.9973, 229.1853)
  line L101 (-94.31, 205.3171) -> (-89.426, 215.2889)
  line L102 (-82.5896, 169.1974) -> (-90.2501, 175.6253)
  line L103 (-90.2501, 175.6253) -> (-101.2909, 174.4464)
  line L104 (-81.8334, 158.1196) -> (-101.2909, 174.4464)
  line L105 (-81.8334, 158.1196) -> (-82.5896, 169.1974)
  line L106 (-53.6234, 132.6992) -> (-63.4715, 134.4357)
  line L107 (-63.4715, 134.4357) -> (-72.4437, 127.8943)
  line L108 (-47.4296, 123.4837) -> (-72.4437, 127.8943)
  line L109 (-47.4296, 123.4837) -> (-53.6234, 132.6992)
  line L110 (-10.2889, 115.574) -> (-19.6858, 112.1538)
  line L111 (-19.6858, 112.1538) -> (-24.1853, 102.0027)
  line L112 (-0.3171, 110.69) -> (-24.1853, 102.0027)
  line L113 (-0.3171, 110.69) -> (-10.2889, 115.574)
  line L114 (35.8026, 122.4104) -> (29.3747, 114.7499)
  line L115 (29.3747, 114.7499) -> (30.5536, 103.7091)
  line L116 (46.8804, 123.1666) -> (30.5536, 103.7091)
  line L117 (46.8804, 123.1666) -> (35.8026, 122.4104)
  line L118 (72.3008, 151.3766) -> (70.5643, 141.5285)
  line L119 (70.5643, 141.5285) -> (77.1057, 132.5563)
  line L120 (81.5163, 157.5704) -> (77.1057, 132.5563)
  line L121 (81.5163, 157.5704) -> (72.3008, 151.3766)
  line L122 (89.426, 194.7111) -> (92.8462, 185.3142)
  line L123 (92.8462, 185.3142) -> (102.9973, 180.8147)
  line L124 (94.31, 204.6829) -> (102.9973, 180.8147)
  line L125 (94.31, 204.6829) -> (89.426, 194.7111)
  line L126 (82.5896, 240.8026) -> (90.2501, 234.3747)
  line L127 (90.2501, 234.3747) -> (101.2909, 235.5536)
  line L128 (81.8334, 251.8804) -> (101.2909, 235.5536)
  line L129 (81.8334, 251.8804) -> (82.5896, 240.8026)
  line L130 (53.6234, 277.3008) -> (63.4715, 275.5643)
  line L131 (63.4715, 275.5643) -> (72.4437, 282.1057)
  line L132 (47.4296, 286.5163) -> (72.4437, 282.1057)
  line L133 (47.4296, 286.5163) -> (53.6234, 277.3008)
  line L134 (-36.5155, 261.714) -> (-44.2419, 253.7395)
  line L135 (-35.6291, 236.3295) -> (-36.5155, 261.714)
  line L136 (-43.8929, 243.7456) -> (-35.6291, 236.3295)
  line L137 (-44.2419, 253.7395) -> (-43.8929, 243.7456)
  line L138 (-65.2222, 187.7973) -> (-60.0256, 177.9848)
  line L139 (-40.8061, 180.7961) -> (-65.2222, 187.7973)
  line L140 (-50.4129, 175.2284) -> (-40.8061, 180.7961)
  line L141 (-60.0256, 177.9848) -> (-50.4129, 175.2284)
  line L142 (-3.794, 137.6541) -> (7.1441, 139.5641)
  line L143 (10.4095, 158.7116) -> (-3.794, 137.6541)
  line L144 (12.736, 147.8545) -> (10.4095, 158.7116)
  line L145 (7.1441, 139.5641) -> (12.736, 147.8545)
  line L146 (62.8774, 180.5807) -> (64.4408, 191.5736)
  line L147 (47.2396, 200.5961) -> (62.8774, 180.5807)
  line L148 (58.2842, 199.4537) -> (47.2396, 200.5961)
  line L149 (64.4408, 191.5736) -> (58.2842, 199.4537)
  point P0 (24.1853, 307.9973)
  dimension "d96" = 360
  dimension "d98" = 360
extrude "Extrude21" cut sketch "Sketch13" against normal up to surface (127 mm away) contours L76 L77 L78 L82 | L83 L84 L88 L89 | L90 L91 L92 L93 | L94 L95 L96 L97 | L98 L99 L100 L101 | L102 L103 L104 L105 | L106 L107 L108 L109 | L110 L111 L112 L113 | L114 L115 L116 L117 | L118 L119 L120 L121 | L122 L123 L124 L125 | L126 L127 L128 L129 | L130 L131 L132 L133 | L134 L135 L136 L137 | L138 L139 L140 L141 | L142 L143 L144 L145 | L146 L147 L148 L149 bodies 27 28 29 30 31 32 33 34 35 36 37 38 39 40 41 42 43
extrude "Extrude11" add sketch "Sketch8" along normal blind 127 separate body contours L147 L150 L151 L152 | L20 L21 L23 L24 L189 L190 L191 L194 L203 L204 L205 L208 L217 L218 L219 L222 L231 L232 L233 L236 L245 L246 L259 L260 L261 L262 L263 L264 L265 L266 L267 L268 L269 L270 L271 L272 L273 L274 L275 | L263 L264 L275 makes body 44 at (-12.4379, 206.2446, 239.6667) makes body 45 at (-87.2502, 223.9299, 239.6667)
move_body "Move1" bodies 7 to x (1, 0, 0) y (0, 1, 0) z (0, 0, 1) at (0, 0, -75)
combine "Combine1" operation cut target body 7 tool bodies 4 keep tools
sketch "Sketch9" plane through (0, 0, 282) normal (0, 0, 1) x (1, 0, 0)
  line L0 (-24.1771, 293.6657) -> (10, 289)
  line L1 (10, 289) -> (-3.6921, 295.7061)
  line L2 (-3.6921, 295.7061) -> (-14.7788, 326.1666)
  line L3 (-14.7788, 326.1666) -> (18.4863, 338.2741)
  line L4 (18.4863, 338.2741) -> (29.573, 307.8136)
  line L5 (29.573, 307.8136) -> (23.3949, 293.8753)
  line L6 (23.3949, 293.8753) -> (50.6603, 272.7461)
  line L7 (50.6603, 272.7461) -> (42.1556, 285.3999)
  line L8 (42.1556, 285.3999) -> (47.7845, 317.3227)
  line L9 (47.7845, 317.3227) -> (82.6467, 311.1756)
  line L10 (82.6467, 311.1756) -> (77.0178, 279.2527)
  line L11 (77.0178, 279.2527) -> (64.6982, 270.2709)
  line L12 (64.6982, 270.2709) -> (77.7461, 238.3397)
  line L13 (77.7461, 238.3397) -> (76.7078, 253.5505)
  line L14 (76.7078, 253.5505) -> (97.5439, 278.3821)
  line L15 (97.5439, 278.3821) -> (124.6619, 255.6274)
  line L16 (124.6619, 255.6274) -> (103.8257, 230.7958)
  line L17 (103.8257, 230.7958) -> (88.6657, 229.1771)
  line L18 (88.6657, 229.1771) -> (84, 195)
  line L19 (84, 195) -> (90.7061, 208.6921)
  line L20 (90.7061, 208.6921) -> (121.1666, 219.7788)
  line L21 (121.1666, 219.7788) -> (133.2741, 186.5137)
  line L22 (133.2741, 186.5137) -> (102.8136, 175.427)
  line L23 (102.8136, 175.427) -> (88.8753, 181.6051)
  line L24 (88.8753, 181.6051) -> (67.7461, 154.3397)
  line L25 (67.7461, 154.3397) -> (80.3999, 162.8444)
  line L26 (80.3999, 162.8444) -> (112.3227, 157.2155)
  line L27 (112.3227, 157.2155) -> (106.1756, 122.3533)
  line L28 (106.1756, 122.3533) -> (74.2527, 127.9822)
  line L29 (74.2527, 127.9822) -> (65.2709, 140.3018)
  line L30 (65.2709, 140.3018) -> (33.3397, 127.2539)
  line L31 (33.3397, 127.2539) -> (48.5505, 128.2922)
  line L32 (48.5505, 128.2922) -> (73.3821, 107.4561)
  line L33 (73.3821, 107.4561) -> (50.6274, 80.3381)
  line L34 (50.6274, 80.3381) -> (25.7958, 101.1743)
  line L35 (25.7958, 101.1743) -> (24.1771, 116.3343)
  line L36 (24.1771, 116.3343) -> (-10, 121)
  line L37 (-10, 121) -> (3.6921, 114.2939)
  line L38 (3.6921, 114.2939) -> (14.7788, 83.8334)
  line L39 (14.7788, 83.8334) -> (-18.4863, 71.7259)
  line L40 (-18.4863, 71.7259) -> (-29.573, 102.1864)
  line L41 (-29.573, 102.1864) -> (-23.3949, 116.1247)
  line L42 (-23.3949, 116.1247) -> (-50.6603, 137.2539)
  line L43 (-50.6603, 137.2539) -> (-42.1556, 124.6001)
  line L44 (-42.1556, 124.6001) -> (-47.7845, 92.6773)
  line L45 (-47.7845, 92.6773) -> (-82.6467, 98.8244)
  line L46 (-82.6467, 98.8244) -> (-77.0178, 130.7473)
  line L47 (-77.0178, 130.7473) -> (-64.6982, 139.7291)
  line L48 (-64.6982, 139.7291) -> (-77.7461, 171.6603)
  line L49 (-77.7461, 171.6603) -> (-76.7078, 156.4495)
  line L50 (-76.7078, 156.4495) -> (-97.5439, 131.6179)
  line L51 (-97.5439, 131.6179) -> (-124.6619, 154.3726)
  line L52 (-124.6619, 154.3726) -> (-103.8257, 179.2042)
  line L53 (-103.8257, 179.2042) -> (-88.6657, 180.8229)
  line L54 (-88.6657, 180.8229) -> (-84, 215)
  line L55 (-84, 215) -> (-90.7061, 201.3079)
  line L56 (-90.7061, 201.3079) -> (-121.1666, 190.2212)
  line L57 (-121.1666, 190.2212) -> (-133.2741, 223.4863)
  line L58 (-133.2741, 223.4863) -> (-102.8136, 234.573)
  line L59 (-102.8136, 234.573) -> (-88.8753, 228.3949)
  line L60 (-88.8753, 228.3949) -> (-67.7461, 255.6603)
  line L61 (-67.7461, 255.6603) -> (-80.3999, 247.1556)
  line L62 (-80.3999, 247.1556) -> (-112.3227, 252.7845)
  line L63 (-112.3227, 252.7845) -> (-106.1756, 287.6467)
  line L64 (-106.1756, 287.6467) -> (-74.2527, 282.0178)
  line L65 (-74.2527, 282.0178) -> (-65.2709, 269.6982)
  line L66 (-65.2709, 269.6982) -> (-33.3397, 282.7461)
  line L67 (-33.3397, 282.7461) -> (-48.5505, 281.7078)
  line L68 (-48.5505, 281.7078) -> (-73.3821, 302.5439)
  line L69 (-73.3821, 302.5439) -> (-50.6274, 329.6619)
  line L70 (-50.6274, 329.6619) -> (-25.7958, 308.8257)
  line L71 (-25.7958, 308.8257) -> (-24.1771, 293.6657)
  line L72 (-172, 377) -> (-172, 33)
  line L73 (-172, 33) -> (172, 33)
  line L74 (172, 33) -> (172, 377)
  line L75 (172, 377) -> (-172, 377)
sketch "Sketch10" plane through (0, 0, -100) normal (0, 0, 1) x (1, 0, 0)
  circle A0 centre (0, 205) radius 100
  line L0 (-145, 0) -> (-145, 30)
  line L1 (-145, 30) -> (-145, 0)
  line L2 (145, 0) -> (145, 30)
  line L3 (145, 30) -> (145, 0)
  line L4 (-145, 30) -> (145, 30)
  line L5 (145, 0) -> (-145, 0)
extrude "Extrude12" add sketch "Sketch10" against normal blind 30 contours L0 L1 L2 L3 L4 L5 bodies 1
sketch "Sketch11" plane through (0, 0, -100) normal (0, 0, 1) x (1, 0, 0)
  circle A0 centre (0, 205) radius 100
  line L0 (-145, 30) -> (-25, 30)
  line L1 (25, 30) -> (145, 30)
  line L2 (135, 30) -> (98.2461, 223.647)
  line L3 (-135, 30) -> (-98.2461, 223.647)
  line L4 (-47.2619, 116.8733) -> (-63.7503, 30)
  line L5 (47.2619, 116.8733) -> (63.7503, 30)
  dimension "d64" = 10
  dimension "d65" = 70
  dimension "d66" = 70
  measures "d64" distance of L1.end L2.start
  measures "d65" distance of L3 L4
  measures "d66" distance of L2 L5
extrude "Extrude13" add sketch "Sketch11" against normal up to surface (300 mm away) separate body contours A0 L1 L2 L5 | A0 L0 L3 L4 makes body 46 at (122.7487, 94.549, -200) makes body 47 at (-122.7487, 94.549, -200)
shell "Shell2" thickness 3 removed faces 4 at (55.3071, 121.6866, -300) at (122.7487, 94.549, -200) at (-122.7487, 94.549, -200) at (-55.3071, 121.6866, -300) on bodies 46 47
sketch "Sketch12" plane through (0, 0, 0) normal (0, -1, 0) x (1, 0, 0)
  line L0 (145, -130) -> (145, -370)
  line L1 (-25, -370) -> (-145, -370)
  line L2 (25, -370) -> (25, -130)
  line L3 (25, -130) -> (145, -130)
  line L4 (-25, -130) -> (-25, -370)
  line L5 (-145, -100) -> (-145, 370)
  line L6 (-145, -130) -> (-25, -130)
  line L7 (145, -100) -> (25, -100)
  line L8 (25, -100) -> (25, 370)
  line L9 (25, 370) -> (145, 370)
  line L10 (145, 370) -> (145, -100)
  line L11 (-145, -400) -> (145, -400)
  line L12 (175, -370) -> (175, 370)
  line L13 (145, 400) -> (-145, 400)
  line L14 (-175, 370) -> (-175, -370)
  line L15 (-25, -100) -> (-145, -100)
  line L16 (-145, 370) -> (-25, 370)
  line L17 (-25, 370) -> (-25, -100)
  line L18 (135, -100) -> (135, -400)
  line L19 (-135, -100) -> (-135, -400)
  circle A0 centre (-120, -115) radius 5
  circle A1 centre (119.4306, -115) radius 5
  circle A2 centre (119.4306, -385) radius 5
  circle A3 centre (-120, -385) radius 5
  line L20 (134.4306, -397) -> (134.4306, -103)
  line L21 (145, -370) -> (175, -370)
  line L22 (175, 370) -> (145, 370)
  line L23 (145, 370) -> (145, 400)
  line L24 (-145, 400) -> (-145, 370)
  line L25 (-145, 370) -> (-175, 370)
  line L26 (-175, -370) -> (-145, -370)
  line L27 (-145, -370) -> (-145, -130)
  line L28 (-145, -370) -> (-145, -400)
  line L29 (145, -400) -> (145, -370)
  line L30 (145, -370) -> (25, -370)
  dimension "d70" = 15
  dimension "d71" = 15
  dimension "d72" = 15
  dimension "d73" = 15
  dimension "d74" = 10
  measures "d70" distance of L15 A0.centre
  measures "d71" distance of L19 A0.centre
  measures "d72" distance of A1.centre L20
  measures "d73" distance of L11 A3.centre
  measures "d74" diameter of A3
extrude "Extrude14" cut sketch "Sketch12" against normal blind 60 contours A0 | A1 | A2 | A3 bodies 1 46 47
extrude "Extrude15" cut sketch "Sketch9" along normal blind 2 contours L0 L1 L2 L3 L4 L5 L6 L7 L8 L9 L10 L11 L12 L13 L14 L15 L16 L17 L18 L19 L20 L21 L22 L23 L24 L25 L26 L27 L28 L29 L30 L31 L32 L33 L34 L35 L36 L37 L38 L39 L40 L41 L42 L43 L44 L45 L46 L47 L48 L49 L50 L51 L52 L53 L54 L55 L56 L57 L58 L59 L60 L61 L62 L63 L64 L65 L66 L67 L68 L69 L70 L71 | L72 L73 L74 L75 bodies 6
extrude "Extrude16" cut 1 faces at (57.3333, 33, 251) along direction (0, -1, 0) blind 2 on bodies 6 bodies 6
extrude "Extrude17" cut 1 faces at (172, 146.3333, 251) along direction (1, 0, 0) blind 2 on bodies 6 bodies 6
extrude "Extrude18" cut 1 faces at (-56.6667, 377, 218) along direction (0, 1, 0) blind 2 on bodies 6 bodies 6
extrude "Extrude20" cut 1 faces at (-172, 263, 218) along direction (-1, 0, 0) blind 2 on bodies 6 bodies 6
sketch "Sketch15" plane through (0, 0, 282) normal (0, 0, 1) x (1, 0, 0)
  line L0 (-24.1771, 293.6657) -> (10, 289)
  line L1 (10, 289) -> (-3.6921, 295.7061)
  line L2 (-3.6921, 295.7061) -> (-14.7788, 326.1666)
  line L3 (-14.7788, 326.1666) -> (18.4863, 338.2741)
  line L4 (18.4863, 338.2741) -> (29.573, 307.8136)
  line L5 (29.573, 307.8136) -> (23.3949, 293.8753)
  line L6 (23.3949, 293.8753) -> (50.6603, 272.7461)
  line L7 (50.6603, 272.7461) -> (42.1556, 285.3999)
  line L8 (42.1556, 285.3999) -> (47.7845, 317.3227)
  line L9 (47.7845, 317.3227) -> (82.6467, 311.1756)
  line L10 (82.6467, 311.1756) -> (77.0178, 279.2527)
  line L11 (77.0178, 279.2527) -> (64.6982, 270.2709)
  line L12 (64.6982, 270.2709) -> (77.7461, 238.3397)
  line L13 (77.7461, 238.3397) -> (76.7078, 253.5505)
  line L14 (76.7078, 253.5505) -> (97.5439, 278.3821)
  line L15 (97.5439, 278.3821) -> (124.6619, 255.6274)
  line L16 (124.6619, 255.6274) -> (103.8257, 230.7958)
  line L17 (103.8257, 230.7958) -> (88.6657, 229.1771)
  line L18 (88.6657, 229.1771) -> (84, 195)
  line L19 (84, 195) -> (90.7061, 208.6921)
  line L20 (90.7061, 208.6921) -> (121.1666, 219.7788)
  line L21 (121.1666, 219.7788) -> (133.2741, 186.5137)
  line L22 (133.2741, 186.5137) -> (102.8136, 175.427)
  line L23 (102.8136, 175.427) -> (88.8753, 181.6051)
  line L24 (88.8753, 181.6051) -> (67.7461, 154.3397)
  line L25 (67.7461, 154.3397) -> (80.3999, 162.8444)
  line L26 (80.3999, 162.8444) -> (112.3227, 157.2155)
  line L27 (112.3227, 157.2155) -> (106.1756, 122.3533)
  line L28 (106.1756, 122.3533) -> (74.2527, 127.9822)
  line L29 (74.2527, 127.9822) -> (65.2709, 140.3018)
  line L30 (65.2709, 140.3018) -> (33.3397, 127.2539)
  line L31 (33.3397, 127.2539) -> (48.5505, 128.2922)
  line L32 (48.5505, 128.2922) -> (73.3821, 107.4561)
  line L33 (73.3821, 107.4561) -> (50.6274, 80.3381)
  line L34 (50.6274, 80.3381) -> (25.7958, 101.1743)
  line L35 (25.7958, 101.1743) -> (24.1771, 116.3343)
  line L36 (24.1771, 116.3343) -> (-10, 121)
  line L37 (-10, 121) -> (3.6921, 114.2939)
  line L38 (3.6921, 114.2939) -> (14.7788, 83.8334)
  line L39 (14.7788, 83.8334) -> (-18.4863, 71.7259)
  line L40 (-18.4863, 71.7259) -> (-29.573, 102.1864)
  line L41 (-29.573, 102.1864) -> (-23.3949, 116.1247)
  line L42 (-23.3949, 116.1247) -> (-50.6603, 137.2539)
  line L43 (-50.6603, 137.2539) -> (-42.1556, 124.6001)
  line L44 (-42.1556, 124.6001) -> (-47.7845, 92.6773)
  line L45 (-47.7845, 92.6773) -> (-82.6467, 98.8244)
  line L46 (-82.6467, 98.8244) -> (-77.0178, 130.7473)
  line L47 (-77.0178, 130.7473) -> (-64.6982, 139.7291)
  line L48 (-64.6982, 139.7291) -> (-77.7461, 171.6603)
  line L49 (-77.7461, 171.6603) -> (-76.7078, 156.4495)
  line L50 (-76.7078, 156.4495) -> (-97.5439, 131.6179)
  line L51 (-97.5439, 131.6179) -> (-124.6619, 154.3726)
  line L52 (-124.6619, 154.3726) -> (-103.8257, 179.2042)
  line L53 (-103.8257, 179.2042) -> (-88.6657, 180.8229)
  line L54 (-88.6657, 180.8229) -> (-84, 215)
  line L55 (-84, 215) -> (-90.7061, 201.3079)
  line L56 (-90.7061, 201.3079) -> (-121.1666, 190.2212)
  line L57 (-121.1666, 190.2212) -> (-133.2741, 223.4863)
  line L58 (-133.2741, 223.4863) -> (-102.8136, 234.573)
  line L59 (-102.8136, 234.573) -> (-88.8753, 228.3949)
  line L60 (-88.8753, 228.3949) -> (-67.7461, 255.6603)
  line L61 (-67.7461, 255.6603) -> (-80.3999, 247.1556)
  line L62 (-80.3999, 247.1556) -> (-112.3227, 252.7845)
  line L63 (-112.3227, 252.7845) -> (-106.1756, 287.6467)
  line L64 (-106.1756, 287.6467) -> (-74.2527, 282.0178)
  line L65 (-74.2527, 282.0178) -> (-65.2709, 269.6982)
  line L66 (-65.2709, 269.6982) -> (-33.3397, 282.7461)
  line L67 (-33.3397, 282.7461) -> (-48.5505, 281.7078)
  line L68 (-48.5505, 281.7078) -> (-73.3821, 302.5439)
  line L69 (-73.3821, 302.5439) -> (-50.6274, 329.6619)
  line L70 (-50.6274, 329.6619) -> (-25.7958, 308.8257)
  line L71 (-25.7958, 308.8257) -> (-24.1771, 293.6657)
  line L72 (-172, 377) -> (-172, 33)
  line L73 (-172, 33) -> (172, 33)
  line L74 (172, 33) -> (172, 377)
  line L75 (172, 377) -> (-172, 377)
  line L76 (145, 30) -> (145, 0)
  line L77 (145, 0) -> (175, 0)
  line L78 (175, 0) -> (175, 30)
  line L79 (175, 30) -> (145, 30)
  line L80 (25, 30) -> (-25, 30)
  line L81 (-25, 30) -> (-25, 0)
  line L82 (-25, 0) -> (25, 0)
  line L83 (25, 0) -> (25, 30)
  line L84 (-145, 30) -> (-175, 30)
  line L85 (-175, 30) -> (-175, 0)
  line L86 (-175, 0) -> (-145, 0)
  line L87 (-145, 0) -> (-145, 30)
  line L88 (142, 33) -> (142, -3)
  line L89 (142, -3) -> (178, -3)
  line L90 (178, -3) -> (178, 33)
  line L91 (178, 33) -> (142, 33)
  dimension "d108" = 3
extrude "Extrude23" add sketch "Sketch15" against normal up to surface (127 mm away) contours L73 L88 L89 L90 L91 bodies 9
mirror "Mirror1" about plane through (0, 0, 0) normal (1, 0, 0) of "Extrude23"
delete_body "RemoveBody1" bodies 21
delete_body "RemoveBody2" bodies 28
delete_body "RemoveBody3" bodies 26
delete_body "RemoveBody4" bodies 27
delete_body "RemoveBody5" bodies 19
delete_body "RemoveBody6" bodies 42
delete_body "RemoveBody7" bodies 29
delete_body "RemoveBody8" bodies 39
delete_body "RemoveBody9" bodies 43
delete_body "RemoveBody10" bodies 36
delete_body "RemoveBody11" bodies 24
delete_body "RemoveBody12" bodies 40
delete_body "RemoveBody13" bodies 11
delete_body "RemoveBody14" bodies 41
delete_body "RemoveBody15" bodies 35
delete_body "RemoveBody16" bodies 31
delete_body "RemoveBody17" bodies 22
delete_body "RemoveBody18" bodies 17
delete_body "RemoveBody19" bodies 33
delete_body "RemoveBody20" bodies 14
delete_body "RemoveBody21" bodies 37
delete_body "RemoveBody22" bodies 34
delete_body "RemoveBody23" bodies 10
delete_body "RemoveBody24" bodies 15
delete_body "RemoveBody25" bodies 12
delete_body "RemoveBody26" bodies 20
delete_body "RemoveBody27" bodies 16
delete_body "RemoveBody28" bodies 25
delete_body "RemoveBody29" bodies 30
delete_body "RemoveBody30" bodies 13
delete_body "RemoveBody31" bodies 7